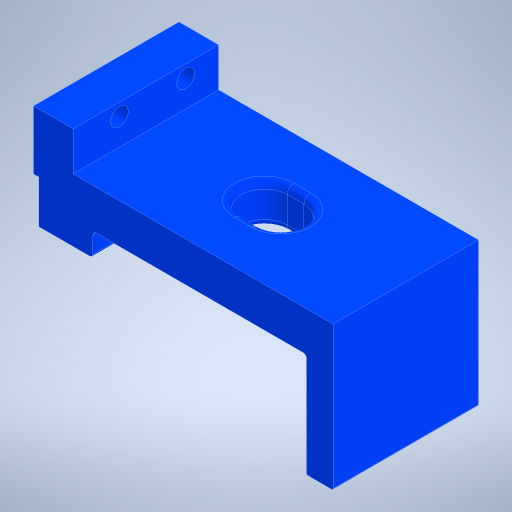
# Autodesk Inventor part: mount_bracket item_5_withhole
Saved by Autodesk Inventor 2023.4 (Build 274418000, 418)
## iProperties
Created: 2022-05-25
Part Number: mount_bracket item_5_withhole
Material: Generic
Document SubType Name: Modeling
Designer: SB13FLLT004
Density: 1 g/cm^3
Appearance: Default(1)
Author: SB13FLLT004
Autodesk Inventor part; units mm, degrees
ref_plane "YZ Plane" through (0, 0, 0) normal (1, 0, 0) x (0, 1, 0)
ref_plane "XZ Plane" through (0, 0, 0) normal (0, 1, 0) x (-1, 0, 0)
ref_plane "XY Plane" through (0, 0, 0) normal (0, 0, 1) x (1, 0, 0)
derived "main_manifold_8v_v02.ipt"
sketch "Sketch:MM: main inlet" plane through (0, 0, 0) normal (1, 0, 0) x (0, 1, 0)
  line L0 (20.32, 0) -> (0, 0)
  line L1 (0, 0) -> (0, -27.94)
  line L2 (0, -27.94) -> (20.32, -27.94)
  line L3 (20.32, -27.94) -> (20.32, 0)
  point P0 (13.97, -15.24)
sketch "Sketch:MM: mounting screws:1" plane through (0, 0, 0) normal (-1, 0, 0) x (0, 0, 1)
  line L0 (-27.94, 0) -> (-27.94, 16.256)
  line L1 (-21.59, 5.08) -> (-8.89, 5.08) construction
  point P0 (0, 0)
  point P1 (-15.24, 13.97)
  point P2 (-15.24, 5.08)
sketch "Sketch: reference" plane through (0, 0, 0) normal (0, 0, 1) x (1, 0, 0)
  line L0 (-24.765, -0.4572) -> (-2.159, -0.4572)
  line L1 (-2.159, -0.4572) -> (-2.159, -4.2672)
  line L2 (-2.159, -4.2672) -> (-24.765, -4.2672)
  line L3 (-24.765, -4.2672) -> (-24.765, -0.4572)
  line L4 (-24.765, 20.32) -> (0, 20.32)
  line L5 (0, 0) -> (-24.765, 0)
  line L6 (-24.765, 0) -> (-24.765, 20.32)
  line L7 (0, 20.32) -> (0, 0) projected
  line L8 (-10.6362, -4.2672) -> (-10.6362, -8.8392)
  line L9 (-10.6362, -8.8392) -> (-1.016, -8.8392)
  line L10 (-1.016, -8.8392) -> (-1.016, -25.2984)
  dimension "d43" = 3.81
  dimension "d45" = 0.4572
  dimension "d47" = 22.606
  dimension "d48" = 2.159
  dimension "d49" = 4.572
  dimension "d50" = 1.016
  dimension "d51" = 8.4772
  constraints: 20 end point, 9 perpendicular, 1 coincident, 1 collinear, 1 point on line
  measures "d43" distance of L0.end L1.end
  measures "d45" distance between parallel lines of L0 L5
  measures "d47" distance of L1.end L2.end
  measures "d48" distance between parallel lines of L7 L1
  measures "d49" distance of L8.start L8.end
  measures "d50" distance between parallel lines of L10 L7
  measures "d51" distance between parallel lines of L8 L1
sketch "Sketch: side profile" plane through (0, 0, 0) normal (0, 0, 1) x (1, 0, 0)
  line L0 (11.938, -7.62) -> (51.938, -7.62) construction
  line L1 (51.938, -7.62) -> (51.938, -47.62) construction
  line L2 (51.938, -47.62) -> (11.938, -47.62) construction
  line L3 (11.938, -47.62) -> (11.938, -7.62) construction
  line L4 (11.43, -12.065) -> (1.016, -12.065)
  line L5 (1.016, -12.065) -> (1.016, 0)
  line L6 (1.016, 0) -> (57.526, 0)
  line L7 (57.526, 0) -> (57.526, -27.62)
  line L8 (52.446, -27.62) -> (52.446, -7.62)
  line L9 (52.446, -7.62) -> (11.43, -7.62)
  line L10 (11.43, -7.62) -> (11.43, -12.065)
  line L11 (11.43, -8.89) -> (11.938, -8.89) construction
  line L12 (52.446, -8.89) -> (51.938, -8.89) construction
  line L13 (0, -3.81) -> (0, 0)
  line L14 (0, 0) -> (1.016, 0)
  line L15 (1.016, -7.62) -> (11.43, -7.62)
  line L16 (57.526, -27.62) -> (52.446, -27.62)
  line L17 (0, -3.81) -> (1.016, -3.81)
  line L18 (0, 20.32) -> (0, 0) construction
  line L19 (-2.159, -4.2672) -> (-24.765, -4.2672) construction
  line L20 (-24.765, -0.4572) -> (-2.159, -0.4572) construction
  line L21 (-2.159, -0.4572) -> (-2.159, -4.2672) construction
  line L22 (-24.765, 20.32) -> (0, 20.32) construction
  line L23 (0, 0) -> (-24.765, 0) construction
  line L24 (-1.016, -8.8392) -> (-1.016, -25.2984) construction
  line L25 (-10.6362, -8.8392) -> (-1.016, -8.8392) construction
  line L26 (-10.6362, -4.2672) -> (-10.6362, -8.8392) construction
  line L27 (53.975, 22.4728) -> (53.975, 6.8361) construction
  point P0 (1.016, -5.08)
  point P1 (0, 0)
  point P2 (0, -3.8003)
  point P3 (51.938, -27.62)
  dimension "d1" = 40
  dimension "d2" = 0.508
  dimension "d3" = 7.62
  dimension "d22" = 1.016
  dimension "d25" = 4.445
  dimension "d30" = 1.27
  dimension "d34" = 11.938
  dimension "d52" = 3.81
  dimension "d53" = 53.975
  dimension "d56" = 12.065
  dimension "d64" = 10.414
  dimension "d65" = 11.43
  dimension "d67" = 5.08
  dimension "d68" = 20
  dimension "d69" = 0
  constraints: 38 end point, 12 perpendicular, 6 point on line, 4 horizontal, 3 collinear, 2 equal length, 1 midpoint, 1 parallel
  measures "d1" distance of L0.start L0.end
  measures "d2" distance of L12.start L12.end
  measures "d3" distance between parallel lines of L6 L9
  measures "d22" distance between parallel lines of L13 L5
  measures "d25" distance of L9.end L4.start
  measures "d30" distance between parallel lines of L0 L12
  measures "d34" distance between parallel lines of L13 L3
  measures "d52" distance of L13.start L13.end
  measures "d53" distance between parallel lines of L27 L18
  measures "d56" distance between parallel lines of L4 L6
  measures "d64" distance of L4.start L4.end
  measures "d65" distance between parallel lines of L10 L13
  measures "d67" distance of L7.end L8.start
  measures "d68" distance between parallel lines of L16 L0
  measures "d69" distance from line of L16 point (51.938, -27.62)
sketch "Sketch: MM holes" plane through (0, 0, 0) normal (1, 0, 0) x (0, 1, 0)
  line L0 (20.32, -27.94) -> (20.32, 0) construction
  line L1 (20.32, 0) -> (0, 0) construction
  line L2 (0, -27.94) -> (20.32, -27.94) construction
  line L3 (0, 0) -> (0, -27.94) construction
  circle A0 centre (5.08, -8.89) radius 1.2065 construction
  line L4 (7.493, 0) -> (0, 0)
  line L5 (0, 0) -> (0, -27.94)
  line L6 (0, -27.94) -> (7.493, -27.94)
  line L7 (7.493, -27.94) -> (7.493, 0)
  point P0 (5.08, -21.59)
  dimension "d5" = 2.413
  dimension "d21" = 7.493
  constraints: 8 end point, 3 collinear, 3 perpendicular, 1 centre point, 1 coincident, 1 vertical
  measures "d5" diameter of A0
  measures "d21" distance of L5.end L6.end
extrude "Ex: MM screws" add sketch "Sketch: MM holes" along normal blind 7.62
hole "Hole: MM screws (4-40)" at (0, 5.08, -8.89) at (0, 5.08, -21.59) direction (1, 0, 0) diameter 3.429 end through all
extrude "Ex: side profile" add sketch "Sketch: side profile" against normal up to surface (27.94 mm away) from surface at 0
sketch "Sketch: center hole" plane through (0, 0, 0) normal (0, 1, 0) x (-1, 0, 0)
  arc A0 (-30.3505, -18.415) -> (-30.3505, -9.525) centre (-30.3505, -13.97) ccw
  arc A1 (-33.5255, -9.525) -> (-33.5255, -18.415) centre (-33.5255, -13.97) ccw
  line L0 (-30.3505, -18.415) -> (-33.5255, -18.415)
  line L1 (-33.5255, -9.525) -> (-30.3505, -9.525)
  line L2 (0, -27.94) -> (0, 0) projected
  line L3 (-30.3505, -13.97) -> (-33.5255, -13.97) construction
  line L4 (-11.938, 0) -> (-51.938, 0) construction
  point P0 (0, 0)
  point P1 (0, -13.97)
  point P2 (-31.938, -13.97)
  point P3 (-31.938, 0)
  point P4 (-37.9705, -13.97)
  point P5 (-25.9055, -13.97)
  dimension "d58" = 4.445
  dimension "d62" = 3.175
  dimension "d63" = 12.065
  constraints: 6 end point, 6 point on circle, 4 tangent, 3 midpoint, 2 centre point, 2 coincident, 1 horizontal, 1 horizontal alignment, 1 parallel, 1 vertical alignment
  measures "d58" radius of A0
  measures "d62" distance of L0.start L0.end
  measures "d63" distance of point (-37.97, -13.97) point (-25.905, -13.97)
extrude "Ex: center hole" cut sketch "Sketch: center hole" against normal through all
fillet "Fillet1" radius 0.635 3 edges at (11.43, -7.62, -13.97) (52.446, -7.62, -13.97) (11.43, -12.065, -13.97)
fillet "Fillet2" radius 0.254 2 edges at (52.446, -27.62, -13.97) (57.526, -27.62, -13.97)
fillet "Fillet3" radius 1.27 8 edges at (37.9705, 0, -13.97) (31.938, 0, -9.525) (25.9055, 0, -13.97) (31.938, 0, -18.415) (25.9055, -7.62, -13.97) (31.938, -7.62, -9.525) (37.9705, -7.62, -13.97) (31.938, -7.62, -18.415)
body "Solid1"
